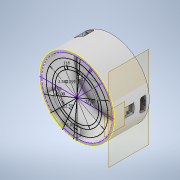
# Autodesk Inventor part: base
Saved by Autodesk Inventor 2020 (Build 240168000, 168)
## iProperties
Created: 2022-01-15
Part Number: base
Material: Generic
Document SubType Name: Modeling
Designer: gamma
Density: 1 g/cm^3
Appearance: Default
Author: gamma
Autodesk Inventor part; units mm, degrees
ref_plane "YZ Plane" through (0, 0, 0) normal (1, 0, 0) x (0, 1, 0)
ref_plane "XZ Plane" through (0, 0, 0) normal (0, 1, 0) x (-1, 0, 0)
ref_plane "XY Plane" through (0, 0, 0) normal (0, 0, 1) x (1, 0, 0)
sketch "Sketch1" plane through (0, 0, 0) normal (0, 0, 1) x (1, 0, 0)
  line L0 (-50.5316, 26.1683) -> (14.4684, 26.1683)
  line L1 (14.4684, 26.1683) -> (14.4684, -3.8317)
  line L2 (14.4684, -3.8317) -> (-50.5316, -3.8317)
  line L3 (-50.5316, -3.8317) -> (-50.5316, 26.1683)
  line L4 (14.4684, 26.1683) -> (10.9684, 26.1683)
  line L5 (14.4684, 22.6683) -> (14.4684, 26.1683)
  line L6 (14.4684, -3.8317) -> (10.9684, -3.8317)
  line L7 (14.4684, -0.3317) -> (14.4684, -3.8317)
  line L8 (-50.5316, 26.1683) -> (-47.0316, 26.1683)
  line L9 (-50.5316, 22.6683) -> (-50.5316, 26.1683)
  line L10 (-50.5316, -3.8317) -> (-47.0316, -3.8317)
  line L11 (-50.5316, -0.3317) -> (-50.5316, -3.8317)
  circle A0 centre (-47.0316, 22.6683) radius 1.25
  circle A1 centre (-47.0316, -0.3317) radius 1.25
  circle A2 centre (10.9684, -0.3317) radius 1.25
  circle A3 centre (10.9684, 22.6683) radius 1.25
  circle A4 centre (-18.0316, 11.1683) radius 37.5
  circle A5 centre (-18.0316, 11.1683) radius 40
  line L12 (14.4684, 26.1683) -> (-39.5316, 26.1683)
  line L13 (-39.5316, 26.1683) -> (-34.0316, 26.1683)
  line L14 (-34.0316, 26.1683) -> (-34.0316, 28.5364)
  line L15 (-39.5316, 26.1683) -> (-45.0316, 26.1683)
  line L16 (-45.0316, 26.1683) -> (-45.0316, 28.5364)
  line L17 (-45.0316, 26.1683) -> (-34.0316, 26.1683)
  line L18 (-34.0316, 26.1683) -> (-34.0316, 51.1683)
  line L19 (-34.0316, 51.1683) -> (-45.0316, 51.1683)
  line L20 (-45.0316, 51.1683) -> (-45.0316, 26.1683)
  line L21 (14.4684, 26.1683) -> (14.4684, 9.2683)
  line L22 (14.4684, 9.2683) -> (14.4684, 16.7683)
  line L23 (14.4684, 9.2683) -> (14.4684, 1.7683)
  line L24 (14.4684, 16.7683) -> (25.9597, 16.7683)
  line L25 (25.9597, 16.7683) -> (25.9597, 1.7683)
  line L26 (25.9597, 1.7683) -> (14.4684, 1.7683)
  line L27 (14.4684, 1.7683) -> (14.4684, 16.7683)
  line L28 (-45.0316, -3.8317) -> (8.9047, -3.8317)
  line L29 (8.9047, -3.8317) -> (8.9047, 2.5262)
  line L30 (8.9047, 2.5262) -> (-45.0316, 2.5262)
  line L31 (-45.0316, 2.5262) -> (-45.0316, -3.8317)
  line L32 (17.6718, 6.5603) -> (17.6718, 11.7374) construction
  line L33 (17.6718, 11.7374) -> (20.8285, 11.7374) construction
  line L34 (20.8285, 11.7374) -> (20.8285, 6.5603) construction
  line L35 (20.8285, 6.5603) -> (17.6718, 6.5603) construction
  line L36 (-3.1073, 38.6557) -> (-8.1073, 38.6557)
  line L37 (-8.1073, 38.6557) -> (-8.1073, 40.6557)
  line L38 (-8.1073, 40.6557) -> (-3.1073, 40.6557)
  line L39 (-3.1073, 40.6557) -> (-3.1073, 38.6557)
  line L40 (-34.4938, 38.6974) -> (-43.1216, 38.6974) construction
  line L41 (-43.1216, 38.6974) -> (-43.1216, 41.864) construction
  line L42 (-43.1216, 41.864) -> (-34.4938, 41.864) construction
  line L43 (-34.4938, 41.864) -> (-34.4938, 38.6974) construction
  spline S0 degree 2 poles (-36.0425, 41.864) (-35.4275, 41.864) (-34.7655, 41.2712) (-34.7655, 40.6981) knots 0 0 0 1 2 2 2
  line L44 (-34.7655, 40.6981) -> (-34.7655, 38.7517)
  line L45 (-34.7655, 38.7517) -> (-35.5313, 38.7517)
  line L46 (-35.5313, 38.7517) -> (-35.5313, 40.6537)
  spline S1 degree 2 poles (-35.5313, 40.6537) (-35.5313, 40.9723) (-35.7708, 41.2835) (-36.0425, 41.2835) knots 0 0 0 1 2 2 2
  spline S2 degree 2 poles (-36.0425, 41.2835) (-36.3068, 41.2835) (-36.5538, 40.9846) (-36.5538, 40.6537) knots 0 0 0 1 2 2 2
  line L47 (-36.5538, 40.6537) -> (-36.5538, 38.7517)
  line L48 (-36.5538, 38.7517) -> (-37.3195, 38.7517)
  line L49 (-37.3195, 38.7517) -> (-37.3195, 40.6957)
  spline S3 degree 2 poles (-37.3195, 40.6957) (-37.3195, 41.2588) (-36.6749, 41.864) (-36.0425, 41.864) knots 0 0 0 1 2 2 2
  spline S4 degree 2 poles (-38.8485, 41.8541) (-38.4977, 41.8541) (-37.9692, 41.7182) (-37.7419, 41.6194) knots 0 0 0 1 2 2 2
  line L50 (-37.7419, 41.6194) -> (-37.7419, 40.8933)
  line L51 (-37.7419, 40.8933) -> (-37.8111, 40.8933)
  spline S5 degree 2 poles (-37.8111, 40.8933) (-38.0408, 41.0884) (-38.5916, 41.2983) (-38.851, 41.2983) knots 0 0 0 1 2 2 2
  spline S6 degree 2 poles (-38.851, 41.2983) (-38.9176, 41.2983) (-39.1325, 41.2687) (-39.1968, 41.2391) knots 0 0 0 1 2 2 2
  spline S7 degree 2 poles (-39.1968, 41.2391) (-39.2758, 41.2045) (-39.3869, 41.0785) (-39.3869, 40.9772) knots 0 0 0 1 2 2 2
  spline S8 degree 2 poles (-39.3869, 40.9772) (-39.3869, 40.8611) (-39.2066, 40.7179) (-39.0831, 40.6858) knots 0 0 0 1 2 2 2
  spline S9 degree 2 poles (-39.0831, 40.6858) (-38.9275, 40.6438) (-38.5743, 40.5721) (-38.4187, 40.5178) knots 0 0 0 1 2 2 2
  spline S10 degree 2 poles (-38.4187, 40.5178) (-38.0655, 40.3943) (-37.7592, 39.9719) (-37.7592, 39.6558) knots 0 0 0 1 2 2 2
  spline S11 degree 2 poles (-37.7592, 39.6558) (-37.7592, 39.2285) (-38.4829, 38.6974) (-39.0263, 38.6974) knots 0 0 0 1 2 2 2
  spline S12 degree 2 poles (-39.0263, 38.6974) (-39.298, 38.6974) (-39.8365, 38.8086) (-40.0489, 38.9024) knots 0 0 0 1 2 2 2
  line L52 (-40.0489, 38.9024) -> (-40.0489, 39.599)
  line L53 (-40.0489, 39.599) -> (-39.9822, 39.599)
  spline S13 degree 2 poles (-39.9822, 39.599) (-39.8118, 39.4532) (-39.3227, 39.2532) (-39.0658, 39.2532) knots 0 0 0 1 2 2 2
  spline S14 degree 2 poles (-39.0658, 39.2532) (-38.9646, 39.2532) (-38.8065, 39.2828) (-38.7176, 39.3223) knots 0 0 0 1 2 2 2
  spline S15 degree 2 poles (-38.7176, 39.3223) (-38.6459, 39.3544) (-38.5422, 39.4829) (-38.5422, 39.5619) knots 0 0 0 1 2 2 2
  spline S16 degree 2 poles (-38.5422, 39.5619) (-38.5422, 39.6805) (-38.7077, 39.8163) (-38.9448, 39.8707) knots 0 0 0 1 2 2 2
  spline S17 degree 2 poles (-38.9448, 39.8707) (-39.098, 39.9052) (-39.382, 39.9719) (-39.545, 40.0287) knots 0 0 0 1 2 2 2
  spline S18 degree 2 poles (-39.545, 40.0287) (-39.8612, 40.1448) (-40.1699, 40.5302) (-40.1699, 40.8463) knots 0 0 0 1 2 2 2
  spline S19 degree 2 poles (-40.1699, 40.8463) (-40.1699, 41.3008) (-39.4561, 41.8541) (-38.8485, 41.8541) knots 0 0 0 1 2 2 2
  spline S20 degree 2 poles (-42.9981, 40.8661) (-42.9981, 41.0933) (-42.8252, 41.4367) (-42.6819, 41.5503) knots 0 0 0 1 2 2 2
  spline S21 degree 2 poles (-42.6819, 41.5503) (-42.509, 41.6861) (-42.099, 41.7997) (-41.7804, 41.7997) knots 0 0 0 1 2 2 2
  line L54 (-41.7804, 41.7997) -> (-40.5627, 41.7997)
  line L55 (-40.5627, 41.7997) -> (-40.5627, 38.7517)
  line L56 (-40.5627, 38.7517) -> (-41.6371, 38.7517)
  spline S22 degree 2 poles (-41.6371, 38.7517) (-41.9731, 38.7517) (-42.3189, 38.8036) (-42.4695, 38.8851) knots 0 0 0 1 2 2 2
  spline S23 degree 2 poles (-42.4695, 38.8851) (-42.635, 38.9716) (-42.7956, 39.268) (-42.7956, 39.4606) knots 0 0 0 1 2 2 2
  spline S24 degree 2 poles (-42.7956, 39.4606) (-42.7956, 39.6829) (-42.5733, 40.0312) (-42.3757, 40.1127) knots 0 0 0 1 2 2 2
  line L57 (-42.3757, 40.1127) -> (-42.3757, 40.1275)
  spline S25 degree 2 poles (-42.3757, 40.1275) (-42.6597, 40.1868) (-42.9981, 40.5549) (-42.9981, 40.8661) knots 0 0 0 1 2 2 2
  spline S26 degree 2 poles (-42.2077, 40.8537) (-42.2077, 40.7105) (-42.0941, 40.5499) (-41.9805, 40.5079) knots 0 0 0 1 2 2 2
  spline S27 degree 2 poles (-41.9805, 40.5079) (-41.9113, 40.4808) (-41.6668, 40.4758) (-41.4642, 40.4758) knots 0 0 0 1 2 2 2
  line L58 (-41.4642, 40.4758) -> (-41.3234, 40.4758)
  line L59 (-41.3234, 40.4758) -> (-41.3234, 41.244)
  line L60 (-41.3234, 41.244) -> (-41.3654, 41.244)
  spline S28 degree 2 poles (-41.3654, 41.244) (-41.6618, 41.244) (-41.8891, 41.2366) (-42.0076, 41.1847) knots 0 0 0 1 2 2 2
  spline S29 degree 2 poles (-42.0076, 41.1847) (-42.1114, 41.1378) (-42.2077, 40.9649) (-42.2077, 40.8537) knots 0 0 0 1 2 2 2
  spline S30 degree 2 poles (-42.0175, 39.6113) (-42.0175, 39.5372) (-41.9409, 39.3816) (-41.8619, 39.347) knots 0 0 0 1 2 2 2
  spline S31 degree 2 poles (-41.8619, 39.347) (-41.7878, 39.3124) (-41.5803, 39.3075) (-41.3753, 39.3075) knots 0 0 0 1 2 2 2
  line L61 (-41.3753, 39.3075) -> (-41.3234, 39.3075)
  line L62 (-41.3234, 39.3075) -> (-41.3234, 39.9546)
  line L63 (-41.3234, 39.9546) -> (-41.4198, 39.9546)
  spline S32 degree 2 poles (-41.4198, 39.9546) (-41.6149, 39.9546) (-41.773, 39.9472) (-41.857, 39.9077) knots 0 0 0 1 2 2 2
  spline S33 degree 2 poles (-41.857, 39.9077) (-41.9484, 39.8633) (-42.0175, 39.7126) (-42.0175, 39.6113) knots 0 0 0 1 2 2 2
  point P0 (0, 0)
  point P1 (8.9047, -3.8317)
  point P2 (18.2712, 1.7683)
  point P3 (20.8483, 1.7683)
  point P4 (21.5745, 16.7683)
  point P5 (19.0479, 16.7683)
  point P6 (-45.0316, 40.681)
  point P7 (-45.0316, 37.1924)
  point P8 (-34.0316, 45.0837)
  point P9 (-34.0316, 47.8289)
  dimension "d0" = 65
  dimension "d1" = 30
  dimension "d14" = 2.5
  dimension "d15" = 2.5
  dimension "d16" = 2.5
  dimension "d17" = 2.5
  dimension "d18" = 75
  dimension "d19" = 80
  dimension "d20" = 54
  dimension "d23" = 16.9
  dimension "d24" = 7.5
  dimension "d25" = 7.5
  dimension "d83" = 5
  dimension "d84" = 2
  constraints: 72 end point, 11 horizontal, 10 parallel, 7 perpendicular, 6 centre point, 5 point on line, 1 coincident, 4 other
  measures "d0" distance of L0.start L0.end
  measures "d1" distance of L0.end L1.end
  measures "d14" diameter of A0
  measures "d15" diameter of A1
  measures "d16" diameter of A2
  measures "d17" diameter of A3
  measures "d18" diameter of A4
  measures "d19" diameter of A5
  measures "d20" distance of L0.end L12.end
  measures "d23" distance of L0.end L21.end
  measures "d24" distance of L21.end L22.end
  measures "d25" distance of L21.end L23.end
  measures "d83" distance of L37.end L38.end
  measures "d84" distance of L36.end L37.end
extrude "Extrusion1" add sketch "Sketch1" against normal blind 2 contours L3 L2 L1 L26 A4 L20 L16 L0 | L0 L1 L2 L29 L30 L31 L3 | L16 L20 A4 S23 S22 L56 L55 L18 L14 L0 | L14 L18 A4 L24 L1 L0 | L20 A5 L18 A4 L55 L54 S21 S20 S25 L57 S24 S23 | A4 L26 A5 L20 | S23 S24 L57 S25 S20 S21 L54 L55 A4 L59 L60 S28 S29 S26 S27 L58 | A4 L58 L59 L55 L56 S22 S23 | L26 L1 L24 A4 | A4 L24 A5 L26 | L31 L30 L29 L2 | L18 A5 L24 A4 | L58 S27 S26 S29 S28 L60 L59 A4 | A4 L59 L58 | A0 | A1 | A2 | A3 | L36 L37 L38 L39 | S0 L44 L45 L46 S1 S2 L47 L48 L49 S3 | S4 L50 L51 S5 S6 S7 S8 S9 S10 S11 S12 L52 L53 S13 S14 S15 S16 S17 S18 S19 | S33 S32 L63 L62 L61 S31 S30
extrude "Extrusion2" add sketch "Sketch1" along normal blind 1.5 contours L0 L1 L2 L29 L30 L31 L3
extrude "Extrusion3" add sketch "Sketch1" along normal blind 5.5 contours A0 | A1 | A2 | A3
extrude "Extrusion4" add sketch "Sketch1" along normal blind 35 contours L20 A5 L18 A4 L55 L54 S21 S20 S25 L57 S24 S23 | A4 L26 A5 L20 | S23 S24 L57 S25 S20 S21 L54 L55 A4 L59 L60 S28 S29 S26 S27 L58 | A4 L24 A5 L26 | L18 A5 L24 A4 | L58 S27 S26 S29 S28 L60 L59 A4
extrude "Extrusion6" cut sketch "Sketch1" along normal blind 12 contours L20 A5 L18 A4 L55 L54 S21 S20 S25 L57 S24 S23 | S23 S24 L57 S25 S20 S21 L54 L55 A4 L59 L60 S28 S29 S26 S27 L58 | L58 S27 S26 S29 S28 L60 L59 A4
fillet "Fillet2" radius 1.5 4 edges at (-34.0316, 46.4563, 12) (-45.0316, 38.9367, 12) (-34.0316, 46.4563, 0) (-45.0316, 38.9367, 0)
sketch "Sketch2" plane through (-18.0316, 11.1683, 35) normal (0, 0, 1) x (1, 0, 0)
  circle A0 centre (0, 0) radius 40 projected
  line L0 (40, 0) -> (-40, 0)
  circle A1 centre (0, 0) radius 32.8
  circle A2 centre (0, 0) radius 26.15
  line L1 (0, 0) -> (-28.2843, -28.2843)
  line L2 (0, 0) -> (0, -40)
  line L3 (0, 0) -> (-15.3073, -36.9552)
  arc A3 (-25.5, 27.4955) -> (-17.5, 33.1662) centre (0, 0) ccw projected
  arc A4 (-14.3506, -34.6455) -> (-26.5165, -26.5165) centre (0, 0) ccw
  line L4 (0, 0) -> (26.5165, 26.5165)
  arc A5 (-25.5, 27.4955) -> (-17.5, 33.1662) centre (0, 0) ccw projected
  line L5 (0, 0) -> (14.3506, 34.6455)
  line L6 (0, 0) -> (0, 37.5)
  line L7 (0, 0) -> (34.6455, 14.3506)
  line L8 (0, 0) -> (-34.6455, -14.3506)
  circle A6 centre (0, 0) radius 37.5 projected
  circle A7 centre (0, 0) radius 23.15
  line L9 (0, 0) -> (-3.4862, -39.8478)
  circle A8 centre (0, 0) radius 40 projected
  line L10 (0, 0) -> (0, 37.5)
  line L11 (0, 0) -> (3.2683, 37.3573)
  point P0 (18.0316, -11.1683)
  point P1 (36.3028, -9.4)
  point P2 (37.0795, 5.6)
  point P3 (0, 37.5)
  point P4 (0, 32.8)
  point P5 (12.552, 30.3032)
  point P6 (0, -37.5)
  point P7 (0, -32.8)
  point P8 (-12.552, -30.3032)
  point P9 (34.6455, 14.3506)
  point P10 (18.4908, 18.4908)
  point P11 (24.1594, 10.0072)
  point P12 (-34.6455, -14.3506)
  point P13 (-18.4908, -18.4908)
  point P14 (-24.1594, -10.0072)
  point P15 (-16.3695, -16.3695)
  point P16 (-21.3878, -8.8591)
  point P17 (16.3695, 16.3695)
  point P18 (21.3878, 8.8591)
  point P19 (2.8587, 32.6752)
  point P20 (3.2683, 37.3573)
  point P21 (0, 37.5)
  point P22 (-2.8587, -32.6752)
  point P23 (-3.2683, -37.3573)
  point P24 (-2.2791, -26.0505)
  point P25 (-10.0072, -24.1594)
  point P26 (2.2791, 26.0505)
  point P27 (10.0072, 24.1594)
  point P28 (0, 26.15)
  point P29 (0, -26.15)
  dimension "d55" = 65.6
  dimension "d56" = 52.3
  dimension "d57" = 45
  dimension "d58" = 22.5
  dimension "d61" = 22.5
  dimension "d62" = 22.5
  dimension "d98" = 3
  dimension "d119" = 5
  constraints: 24 end point, 14 point on circle, 4 centre point, 3 coincident, 3 point on line, 1 horizontal, 1 perpendicular, 1 vertical, 4 other
  measures "d55" diameter of A1
  measures "d56" diameter of A2
  measures "d57" angle of L0 L1
  measures "d58" angle of L1 L3
  measures "d61" angle of L0 L7
  measures "d62" angle of L0 L8
  measures "d98" radial gap between concentric circles of A2 A7
  measures "d119" angle of L2 L9
extrude "Extrusion9" add sketch "Sketch2" against normal blind 5.96 contours A3 L9 A1 L2 | A3 L3 A1 L9 | L6 A3 L11 A1 | L5 A1 L11 A3
extrude "Extrusion10" add sketch "Sketch2" against normal blind 6 contours L7 A1 L4 A3 | L7 A2 L4 A1
chamfer "Chamfer1" distance 7.9375 angle 45 1 edges at (13.1485, 32.0022, 29)
chamfer "Chamfer2" distance 3.302 angle 45 1 edges at (3.7114, 25.6965, 29)
extrude "Extrusion11" add sketch "Sketch2" against normal blind 6 contours A3 L8 A1 L1 | A1 L8 A2 L1
chamfer "Chamfer3" distance 7.9375 angle 45 1 edges at (-49.2117, -9.6656, 29)
chamfer "Chamfer4" distance 3.302 angle 45 1 edges at (-39.7745, -3.3598, 29)
extrude "Extrusion13" add sketch "Sketch1" along normal blind 10 contours L36 L37 L38 L39
fillet "Fillet4" radius 0.762 4 edges at (-8.1073, 39.6557, 0) (-5.6073, 40.6557, 0) (-3.1073, 39.6557, 0) (-5.6073, 38.6557, 0)
extrude "Extrusion14" add sketch "Sketch1" along normal blind 1.5 contours L26 L1 L24 A4 | A4 L24 A5 L26
sketch "Sketch5" plane through (0, 0, 1.5) normal (0, 0, 1) x (1, 0, 0)
  line L0 (14.4684, 1.7683) -> (14.4684, -3.8317) projected
  line L1 (14.4684, 1.7683) -> (26.01, 1.7683)
  line L2 (26.01, 1.7683) -> (26.01, 16.7683)
  line L3 (26.01, 16.7683) -> (14.4684, 16.7683)
  line L4 (14.4684, 16.7683) -> (14.4684, 1.7683)
  line L5 (17.4931, 5.9317) -> (17.4931, 11.7609) construction
  line L6 (17.4931, 11.7609) -> (20.6498, 11.7609) construction
  line L7 (20.6498, 11.7609) -> (20.6498, 5.9317) construction
  line L8 (20.6498, 5.9317) -> (17.4931, 5.9317) construction
  spline S0 degree 2 poles (21.1759, 7.3985) (21.1759, 6.9893) (21.0174, 6.3726) (20.9022, 6.1075) knots 0 0 0 1 2 2 2
  line L9 (20.9022, 6.1075) -> (20.055, 6.1075)
  line L10 (20.055, 6.1075) -> (20.055, 6.1881)
  spline S1 degree 2 poles (20.055, 6.1881) (20.2826, 6.4561) (20.5276, 7.0988) (20.5276, 7.4013) knots 0 0 0 1 2 2 2
  spline S2 degree 2 poles (20.5276, 7.4013) (20.5276, 7.4791) (20.493, 7.7299) (20.4584, 7.8048) knots 0 0 0 1 2 2 2
  spline S3 degree 2 poles (20.4584, 7.8048) (20.4181, 7.897) (20.2711, 8.0267) (20.1529, 8.0267) knots 0 0 0 1 2 2 2
  spline S4 degree 2 poles (20.1529, 8.0267) (20.0175, 8.0267) (19.8504, 7.8163) (19.8129, 7.6722) knots 0 0 0 1 2 2 2
  spline S5 degree 2 poles (19.8129, 7.6722) (19.7639, 7.4907) (19.6803, 7.0786) (19.6169, 6.897) knots 0 0 0 1 2 2 2
  spline S6 degree 2 poles (19.6169, 6.897) (19.4729, 6.485) (18.9801, 6.1276) (18.6112, 6.1276) knots 0 0 0 1 2 2 2
  spline S7 degree 2 poles (18.6112, 6.1276) (18.1127, 6.1276) (17.4931, 6.972) (17.4931, 7.6059) knots 0 0 0 1 2 2 2
  spline S8 degree 2 poles (17.4931, 7.6059) (17.4931, 7.9229) (17.6228, 8.5511) (17.7323, 8.799) knots 0 0 0 1 2 2 2
  line L11 (17.7323, 8.799) -> (18.545, 8.799)
  line L12 (18.545, 8.799) -> (18.545, 8.7212)
  spline S9 degree 2 poles (18.545, 8.7212) (18.3749, 8.5223) (18.1415, 7.9517) (18.1415, 7.652) knots 0 0 0 1 2 2 2
  spline S10 degree 2 poles (18.1415, 7.652) (18.1415, 7.5339) (18.1761, 7.3495) (18.2222, 7.2457) knots 0 0 0 1 2 2 2
  spline S11 degree 2 poles (18.2222, 7.2457) (18.2597, 7.1622) (18.4095, 7.0411) (18.5017, 7.0411) knots 0 0 0 1 2 2 2
  spline S12 degree 2 poles (18.5017, 7.0411) (18.6401, 7.0411) (18.7985, 7.2342) (18.8619, 7.5108) knots 0 0 0 1 2 2 2
  spline S13 degree 2 poles (18.8619, 7.5108) (18.9023, 7.6895) (18.9801, 8.0209) (19.0464, 8.2111) knots 0 0 0 1 2 2 2
  spline S14 degree 2 poles (19.0464, 8.2111) (19.1818, 8.5799) (19.6314, 8.9402) (20.0002, 8.9402) knots 0 0 0 1 2 2 2
  spline S15 degree 2 poles (20.0002, 8.9402) (20.5304, 8.9402) (21.1759, 8.1074) (21.1759, 7.3985) knots 0 0 0 1 2 2 2
  spline S16 degree 2 poles (19.3374, 12.5711) (19.836, 12.5711) (20.6198, 12.1359) (20.8301, 11.8046) knots 0 0 0 1 2 2 2
  spline S17 degree 2 poles (20.8301, 11.8046) (21.0088, 11.5279) (21.1125, 10.8767) (21.1125, 10.5107) knots 0 0 0 1 2 2 2
  line L13 (21.1125, 10.5107) -> (21.1125, 9.3983)
  line L14 (21.1125, 9.3983) -> (17.5565, 9.3983)
  line L15 (17.5565, 9.3983) -> (17.5565, 10.4992)
  spline S18 degree 2 poles (17.5565, 10.4992) (17.5565, 10.8738) (17.6516, 11.5279) (17.8361, 11.8161) knots 0 0 0 1 2 2 2
  spline S19 degree 2 poles (17.8361, 11.8161) (18.0608, 12.1648) (18.8216, 12.5711) (19.3374, 12.5711) knots 0 0 0 1 2 2 2
  spline S20 degree 2 poles (19.3317, 11.6547) (18.9801, 11.6547) (18.4787, 11.4126) (18.3375, 11.1648) knots 0 0 0 1 2 2 2
  spline S21 degree 2 poles (18.3375, 11.1648) (18.2395, 10.9833) (18.2193, 10.5856) (18.2193, 10.309) knots 0 0 0 1 2 2 2
  line L16 (18.2193, 10.309) -> (18.2193, 10.2917)
  line L17 (18.2193, 10.2917) -> (20.4469, 10.2917)
  line L18 (20.4469, 10.2917) -> (20.4469, 10.309)
  spline S22 degree 2 poles (20.4469, 10.309) (20.4469, 10.6087) (20.4267, 11.0207) (20.3085, 11.208) knots 0 0 0 1 2 2 2
  spline S23 degree 2 poles (20.3085, 11.208) (20.1702, 11.4271) (19.6832, 11.6547) (19.3317, 11.6547) knots 0 0 0 1 2 2 2
  point P0 (0, 0)
  constraints: 8 end point, 2 parallel, 1 horizontal, 1 perpendicular, 2 other
extrude "Extrusion15" cut sketch "Sketch5" along normal blind 6 contours L4 L3 L2 L1 | S0 L9 L10 S1 S2 S3 S4 S5 S6 S7 S8 L11 L12 S9 S10 S11 S12 S13 S14 S15 | S16 S17 L13 L14 L15 S18 S19 | S23 S22 L18 L17 L16 S21 S20
extrude "Extrusion16" cut sketch "Sketch5" against normal blind 0.5 contours S0 L9 L10 S1 S2 S3 S4 S5 S6 S7 S8 L11 L12 S9 S10 S11 S12 S13 S14 S15 | S16 S17 L13 L14 L15 S18 S19
fillet "Fillet5" radius 2.286 2 edges at (20.3112, 16.7683, 7.5) (19.5597, 1.7683, 7.5)
extrude "Extrusion17" cut sketch "Sketch1" against normal blind 0.5 contours S23 S24 L57 S25 S20 S21 L54 L55 A4 L59 L60 S28 S29 S26 S27 L58 | A4 L58 L59 L55 L56 S22 S23 | S0 L44 L45 L46 S1 S2 L47 L48 L49 S3 | S4 L50 L51 S5 S6 S7 S8 S9 S10 S11 S12 L52 L53 S13 S14 S15 S16 S17 S18 S19
fillet "Fillet6" radius 0.762 4 edges at (9.7184, 22.6683, 1.5) (9.7184, -0.3317, 1.5) (-48.2816, -0.3317, 1.5) (-48.2816, 22.6683, 1.5)
extrude "Extrusion18" add sketch "Sketch2" against normal blind 2.5 contours L7 A7 L4 A2 | A2 L8 A7 L1
extrude "Extrusion19" add sketch "Sketch2" along normal blind 1.5 contours L7 A7 L4 A2 | A2 L8 A7 L1
chamfer "Chamfer5" distance 0.762 angle 45 4 edges at (1.217, 24.0298, 32.5) (-37.2801, -1.6931, 32.5) (-39.7745, -3.3598, 36.5) (3.7114, 25.6965, 36.5)
ref_plane "Work Plane3" through (21.9684, 11.1683, 35) normal (1, 0, 0) x (0, 1, 0)
sketch "Sketch6" plane through (21.9684, 11.1683, 35) normal (1, 0, 0) x (0, 1, 0)
  line L0 (40, 0) -> (-40, 0) projected
  line L1 (0, 0) -> (0, -16)
  line L2 (-4.825, -20.85) -> (4.825, -20.85)
  line L3 (4.825, -20.85) -> (4.825, -11.15)
  line L4 (4.825, -11.15) -> (-4.825, -11.15)
  line L5 (-4.825, -11.15) -> (-4.825, -20.85)
  line L6 (-4.825, -20.85) -> (4.825, -11.15) construction
  line L7 (4.825, -20.85) -> (-4.825, -11.15) construction
  point P0 (-11.1683, -35)
  dimension "d106" = 16
  dimension "d107" = 9.65
  dimension "d108" = 9.7
  constraints: 14 end point, 3 midpoint, 2 parallel, 1 horizontal, 1 perpendicular, 1 vertical
  measures "d106" distance of L1.start L1.end
  measures "d107" distance of L2.start L2.end
  measures "d108" distance of L3.end L2.end
extrude "Extrusion20" cut sketch "Sketch6" against normal blind 4
ref_plane "Work Plane4" through (19.4684, 11.1683, 14.15) normal (1, 0, 0) x (0, 1, 0)
sketch "Sketch7" plane through (19.4684, 11.1683, 14.15) normal (1, 0, 0) x (0, 1, 0)
  line L0 (14.4849, -0.0211) -> (-4.825, -0.0211)
  line L1 (-4.825, -0.0211) -> (-4.825, -2.0211)
  line L2 (-4.825, -2.0211) -> (14.4849, -2.0211)
  line L3 (14.4849, -2.0211) -> (14.4849, -0.0211)
  line L4 (-4.825, -2.0211) -> (-6.825, -2.0211)
  line L5 (-6.825, -2.0211) -> (-6.825, 2.4048)
  line L6 (-6.825, 2.4048) -> (-4.825, 2.4048)
  line L7 (-4.825, 2.4048) -> (-4.825, -2.0211)
  line L8 (4.83, -2.0211) -> (6.83, -2.0211)
  line L9 (6.83, -2.0211) -> (6.83, 2.5486)
  line L10 (6.83, 2.5486) -> (4.83, 2.5486)
  line L11 (4.83, 2.5486) -> (4.83, -2.0211)
  point P0 (-11.1683, -14.15)
  point P1 (6.83, -2.0211)
  point P2 (4.83, -0.0211)
  point P3 (-4.825, -0.0211)
  dimension "d111" = 2
  dimension "d112" = 2
  dimension "d114" = 2
  dimension "d115" = 4.5697
  constraints: 24 end point, 6 parallel, 3 horizontal, 3 perpendicular, 1 midpoint
  measures "d111" distance of L0.end L1.end
  measures "d112" distance of L5.end L6.end
  measures "d114" distance of L10.end L9.end
  measures "d115" distance of L8.end L9.end
extrude "Extrusion21" add sketch "Sketch7" against normal blind 3 contours L9 L2 L11 L0 | L0 L11 L10 L9 | L11 L2 L1 L0 | L1 L4 L5 L6 L7
fillet "Fillet7" radius 1.397 2 edges at (19.3113, 14.5977, 12.1289) (19.3115, 7.7415, 12.1289)
extrude "Extrusion23" add sketch "Sketch2" against normal blind 6 contours A1 L9 A2 L2 | A1 L11 A2 L6 | A1 L3 A2 L9 | A1 L5 A2 L11
chamfer "Chamfer6" distance 5.08 angle 45 2 edges at (-12.9299, 36.8159, 29) (-23.1332, -14.4792, 29)
fillet "Fillet8" radius 2.286 4 edges at (-18.0316, 43.1833, 29) (-18.0316, 46.3183, 29.04) (-18.0316, -20.8467, 29) (-18.0316, -23.9817, 29.04)
fillet "Fillet9" radius 0.254 4 edges at (-4.5802, 43.6427, 29.04) (-5.78, 40.7463, 29) (-31.4829, -21.306, 29.04) (-30.2832, -18.4097, 29)
sketch "Sketch8" plane through (-18.0316, 11.1683, -2) normal (0, 0, -1) x (-1, 0, 0)
  line L0 (16.6916, 18.2128) -> (-16.4283, 18.2128) construction
  line L1 (-16.4283, 18.2128) -> (-16.4283, 33.2955) construction
  line L2 (-16.4283, 33.2955) -> (16.6916, 33.2955) construction
  line L3 (16.6916, 33.2955) -> (16.6916, 18.2128) construction
  line L4 (8.4762, 23.3998) -> (11.2097, 23.3998)
  line L5 (11.2097, 23.3998) -> (11.2097, 22.5147)
  line L6 (11.2097, 22.5147) -> (10.481, 22.5147)
  line L7 (10.481, 22.5147) -> (10.481, 19.2049)
  line L8 (10.481, 19.2049) -> (11.2097, 19.2049)
  line L9 (11.2097, 19.2049) -> (11.2097, 18.3198)
  line L10 (11.2097, 18.3198) -> (8.4762, 18.3198)
  line L11 (8.4762, 18.3198) -> (8.4762, 19.2049)
  line L12 (8.4762, 19.2049) -> (9.2048, 19.2049)
  line L13 (9.2048, 19.2049) -> (9.2048, 22.5147)
  line L14 (9.2048, 22.5147) -> (8.4762, 22.5147)
  line L15 (8.4762, 22.5147) -> (8.4762, 23.3998)
  line L16 (1.1114, 23.3504) -> (5.4916, 21.5308)
  line L17 (5.4916, 21.5308) -> (5.4916, 20.7816)
  line L18 (5.4916, 20.7816) -> (1.1114, 18.962)
  line L19 (1.1114, 18.962) -> (1.1114, 19.9047)
  line L20 (1.1114, 19.9047) -> (4.1742, 21.1603)
  line L21 (4.1742, 21.1603) -> (1.1114, 22.4077)
  line L22 (1.1114, 22.4077) -> (1.1114, 23.3504)
  spline S0 degree 2 poles (-3.7298, 21.8602) (-3.7298, 22.2348) (-3.454, 22.8482) (-3.1864, 23.0622) knots 0 0 0 1 2 2 2
  spline S1 degree 2 poles (-3.1864, 23.0622) (-2.9188, 23.2763) (-2.1902, 23.5068) (-1.6673, 23.5068) knots 0 0 0 1 2 2 2
  spline S2 degree 2 poles (-1.6673, 23.5068) (-1.0745, 23.5068) (-0.2265, 23.3092) (0.0411, 23.1857) knots 0 0 0 1 2 2 2
  line L23 (0.0411, 23.1857) -> (0.0411, 22.0825)
  line L24 (0.0411, 22.0825) -> (-0.0824, 22.0825)
  spline S3 degree 2 poles (-0.0824, 22.0825) (-0.3624, 22.2595) (-1.1157, 22.5229) (-1.4286, 22.5229) knots 0 0 0 1 2 2 2
  spline S4 degree 2 poles (-1.4286, 22.5229) (-1.6138, 22.5229) (-2.0461, 22.4571) (-2.1943, 22.35) knots 0 0 0 1 2 2 2
  spline S5 degree 2 poles (-2.1943, 22.35) (-2.3095, 22.2636) (-2.4495, 22.0125) (-2.4495, 21.7861) knots 0 0 0 1 2 2 2
  spline S6 degree 2 poles (-2.4495, 21.7861) (-2.4495, 21.5596) (-2.2519, 21.3168) (-2.0872, 21.2591) knots 0 0 0 1 2 2 2
  spline S7 degree 2 poles (-2.0872, 21.2591) (-1.9226, 21.2015) (-1.4656, 21.1891) (-1.2886, 21.1891) knots 0 0 0 1 2 2 2
  line L25 (-1.2886, 21.1891) -> (-1.0704, 21.1891)
  line L26 (-1.0704, 21.1891) -> (-1.0704, 20.2958)
  line L27 (-1.0704, 20.2958) -> (-1.2721, 20.2958)
  spline S8 degree 2 poles (-1.2721, 20.2958) (-1.5027, 20.2958) (-1.8938, 20.2546) (-2.0296, 20.1929) knots 0 0 0 1 2 2 2
  spline S9 degree 2 poles (-2.0296, 20.1929) (-2.1655, 20.127) (-2.3178, 19.8965) (-2.3178, 19.6989) knots 0 0 0 1 2 2 2
  spline S10 degree 2 poles (-2.3178, 19.6989) (-2.3178, 19.5425) (-2.1737, 19.349) (-2.0708, 19.2955) knots 0 0 0 1 2 2 2
  spline S11 degree 2 poles (-2.0708, 19.2955) (-1.9473, 19.2337) (-1.6179, 19.1925) (-1.5027, 19.1925) knots 0 0 0 1 2 2 2
  spline S12 degree 2 poles (-1.5027, 19.1925) (-1.3174, 19.1925) (-0.9263, 19.279) (-0.7452, 19.349) knots 0 0 0 1 2 2 2
  spline S13 degree 2 poles (-0.7452, 19.349) (-0.6011, 19.4025) (-0.2883, 19.5754) (-0.2141, 19.6207) knots 0 0 0 1 2 2 2
  line L28 (-0.2141, 19.6207) -> (-0.1071, 19.6207)
  line L29 (-0.1071, 19.6207) -> (-0.1071, 18.5339)
  spline S14 degree 2 poles (-0.1071, 18.5339) (-0.3706, 18.4227) (-1.2598, 18.2128) (-1.725, 18.2128) knots 0 0 0 1 2 2 2
  spline S15 degree 2 poles (-1.725, 18.2128) (-2.1778, 18.2128) (-2.8447, 18.3692) (-3.0794, 18.5215) knots 0 0 0 1 2 2 2
  spline S16 degree 2 poles (-3.0794, 18.5215) (-3.3387, 18.6821) (-3.5981, 19.1761) (-3.5981, 19.4848) knots 0 0 0 1 2 2 2
  spline S17 degree 2 poles (-3.5981, 19.4848) (-3.5981, 19.9212) (-3.0958, 20.5716) (-2.6842, 20.6663) knots 0 0 0 1 2 2 2
  line L30 (-2.6842, 20.6663) -> (-2.6842, 20.7157)
  spline S18 degree 2 poles (-2.6842, 20.7157) (-2.8653, 20.7404) (-3.2111, 20.8721) (-3.3758, 21.0203) knots 0 0 0 1 2 2 2
  spline S19 degree 2 poles (-3.3758, 21.0203) (-3.5281, 21.1521) (-3.7298, 21.572) (-3.7298, 21.8602) knots 0 0 0 1 2 2 2
  spline S20 degree 2 poles (-8.6863, 23.5068) (-7.6612, 23.5068) (-6.558, 22.5188) (-6.558, 21.5638) knots 0 0 0 1 2 2 2
  line L31 (-6.558, 21.5638) -> (-6.558, 18.3198)
  line L32 (-6.558, 18.3198) -> (-7.8341, 18.3198)
  line L33 (-7.8341, 18.3198) -> (-7.8341, 21.4897)
  spline S21 degree 2 poles (-7.8341, 21.4897) (-7.8341, 22.0207) (-8.2335, 22.5394) (-8.6863, 22.5394) knots 0 0 0 1 2 2 2
  spline S22 degree 2 poles (-8.6863, 22.5394) (-9.1268, 22.5394) (-9.5385, 22.0413) (-9.5385, 21.4897) knots 0 0 0 1 2 2 2
  line L34 (-9.5385, 21.4897) -> (-9.5385, 18.3198)
  line L35 (-9.5385, 18.3198) -> (-10.8146, 18.3198)
  line L36 (-10.8146, 18.3198) -> (-10.8146, 21.5596)
  spline S23 degree 2 poles (-10.8146, 21.5596) (-10.8146, 22.4982) (-9.7402, 23.5068) (-8.6863, 23.5068) knots 0 0 0 1 2 2 2
  line L37 (1.6054, 29.9937) -> (3.8655, 29.9937)
  line L38 (3.8655, 29.9937) -> (3.8655, 29.0469)
  line L39 (3.8655, 29.0469) -> (1.6054, 29.0469)
  line L40 (1.6054, 29.0469) -> (1.6054, 29.9937)
  spline S24 degree 2 poles (-3.5404, 31.4757) (-3.207, 31.6116) (-2.1408, 31.8709) (-1.6221, 31.8709) knots 0 0 0 1 2 2 2
  spline S25 degree 2 poles (-1.6221, 31.8709) (-0.4241, 31.8709) (0.9962, 30.4877) (0.9962, 29.2198) knots 0 0 0 1 2 2 2
  spline S26 degree 2 poles (0.9962, 29.2198) (0.9962, 28.0259) (-0.4241, 26.5851) (-1.6591, 26.5851) knots 0 0 0 1 2 2 2
  spline S27 degree 2 poles (-1.6591, 26.5851) (-2.2972, 26.5851) (-3.0958, 26.828) (-3.5199, 27.0338) knots 0 0 0 1 2 2 2
  line L41 (-3.5199, 27.0338) -> (-3.5199, 28.2276)
  line L42 (-3.5199, 28.2276) -> (-3.4046, 28.2276)
  spline S28 degree 2 poles (-3.4046, 28.2276) (-3.314, 28.1577) (-2.9682, 27.8901) (-2.8035, 27.7995) knots 0 0 0 1 2 2 2
  spline S29 degree 2 poles (-2.8035, 27.7995) (-2.6142, 27.6884) (-2.1119, 27.5319) (-1.832, 27.5319) knots 0 0 0 1 2 2 2
  spline S30 degree 2 poles (-1.832, 27.5319) (-1.5068, 27.5319) (-0.9675, 27.7378) (-0.7576, 27.9477) knots 0 0 0 1 2 2 2
  spline S31 degree 2 poles (-0.7576, 27.9477) (-0.5558, 28.1535) (-0.3212, 28.7834) (-0.3212, 29.1992) knots 0 0 0 1 2 2 2
  spline S32 degree 2 poles (-0.3212, 29.1992) (-0.3212, 30.0884) (-1.2145, 30.9364) (-1.9843, 30.9364) knots 0 0 0 1 2 2 2
  spline S33 degree 2 poles (-1.9843, 30.9364) (-2.0543, 30.9364) (-2.2354, 30.9282) (-2.3054, 30.9241) knots 0 0 0 1 2 2 2
  line L43 (-2.3054, 30.9241) -> (-2.3054, 29.9237)
  line L44 (-2.3054, 29.9237) -> (-1.3215, 29.9237)
  line L45 (-1.3215, 29.9237) -> (-1.3215, 28.9728)
  line L46 (-1.3215, 28.9728) -> (-3.5404, 28.9728)
  line L47 (-3.5404, 28.9728) -> (-3.5404, 31.4757)
  point P0 (-18.0316, -11.1683)
  constraints: 2 other
extrude "Extrusion24" cut sketch "Sketch8" against normal blind 0.5
body "Solid1"
